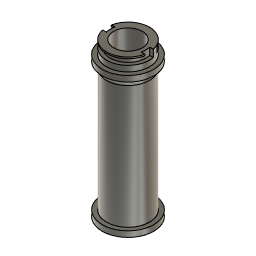
Spool_Holder_Handle_Easier_print_v1 (Autodesk Fusion 360 design; units mm, degrees)
Autodesk Fusion 360 part; units mm, degrees
sketch "Sketch1" plane through (0, 0, 0) normal (0, 0, 1) x (1, 0, 0)
  circle A0 centre (0, 0) radius 18
  dimension "d1" = 36
  constraint coincident A0.centre origin
  measures "d1" diameter of A0
sketch "Sketch2" plane through (0, 0, 0) normal (0, 0, 1) x (1, 0, 0)
  circle A0 centre (0, 0) radius 15
  circle A1 centre (0, 0) radius 13
  constraint coincident A0.centre A1.centre
extrude "Extrude1" add sketch "Sketch1" along normal blind 4
extrude "Extrude2" add sketch "Sketch2" along normal blind 110
sketch "Sketch3" plane through (0, 0, 110) normal (0, 0, 1) x (-1, 0, 0)
  circle A0 centre (0, 0) radius 15
  arc A1 (14.6969, 3) -> (3, 14.6969) centre (0, 0) ccw
  arc A2 (-3, 14.6969) -> (-14.6969, 3) centre (0, 0) ccw
  arc A3 (-14.6969, -3) -> (-3, -14.6969) centre (0, 0) ccw
  arc A4 (3, -14.6969) -> (14.6969, -3) centre (0, 0) ccw
  line L0 (11.619, -3) -> (14.6969, -3)
  arc A5 (11.619, -3) -> (11.619, 3) centre (0, 0) ccw
  arc A6 (3, 11.619) -> (-3, 11.619) centre (0, 0) ccw
  arc A7 (-11.619, 3) -> (-11.619, -3) centre (0, 0) ccw
  arc A8 (-3, -11.619) -> (3, -11.619) centre (0, 0) ccw
  line L1 (-14.6969, -3) -> (-11.619, -3)
  line L2 (14.6969, 3) -> (11.619, 3)
  line L3 (-11.619, 3) -> (-14.6969, 3)
  line L4 (-3, 14.6969) -> (-3, 11.619)
  line L5 (-3, -11.619) -> (-3, -14.6969)
  line L6 (3, -14.6969) -> (3, -11.619)
  line L7 (3, 11.619) -> (3, 14.6969)
  line L8 (8.6603, -5) -> (10.3923, -6)
  line L9 (0, 0) -> (12, 0) construction
  line L10 (-8.6603, -5) -> (-10.3923, -6)
  line L11 (4.8249, -8.3569) -> (6, -10.3923)
  line L12 (-4.8249, -8.3569) -> (-6, -10.3923)
  line L13 (8.6603, 5) -> (10.3923, 6)
  line L14 (-8.6603, 5) -> (-10.3923, 6)
  line L15 (5, 8.6603) -> (6, 10.3923)
  line L16 (-5, 8.6603) -> (-6, 10.3923)
  arc A9 (6, -10.3923) -> (10.3923, -6) centre (0, 0) ccw
  arc A10 (-3, -11.619) -> (3, -11.619) centre (0, 0) ccw
  arc A11 (-10.3923, -6) -> (-6, -10.3923) centre (0, 0) ccw
  arc A12 (-6, 10.3923) -> (-10.3923, 6) centre (0, 0) ccw
  arc A13 (3, 11.619) -> (-3, 11.619) centre (0, 0) ccw
  arc A14 (11.619, -3) -> (11.619, 3) centre (0, 0) ccw
  arc A15 (10.3923, 6) -> (6, 10.3923) centre (0, 0) ccw
  arc A16 (5, 8.6603) -> (-5, 8.6603) centre (0, 0) ccw
  arc A17 (-8.6603, 5) -> (-8.6603, -5) centre (0, 0) ccw
  arc A18 (-4.8249, -8.3569) -> (4.8249, -8.3569) centre (0, 0) ccw
  arc A19 (8.6603, -5) -> (8.6603, 5) centre (0, 0) ccw
  dimension "d6" = 30
  constraint coincident A4.start A1
  constraint perpendicular L1 L4
  constraint perpendicular L2 L4
  constraint concentric A1 A2
  constraint concentric A2 A3
  constraint concentric A3 A4
  constraint collinear L0 L1
  constraint coincident A6.start L6
  constraint concentric A5 A6
  constraint coincident A7.start L2
  constraint concentric A6 A7
  constraint coincident A8.start L4
  constraint concentric A7 A8
  constraint collinear L4 L5
  constraint collinear L6 L7
  constraint concentric A2 A16
  constraint concentric A7 A14
  constraint horizontal L9
  constraint coincident A0.centre A1.centre
  constraint coincident L10.end A14
  constraint coincident L11.end A14
  constraint perpendicular L10 L11
  constraint perpendicular L8 L12
  constraint coincident L13.end A14
  constraint parallel L10 L13
  constraint perpendicular L14 L15
  constraint coincident L16.end A14
  constraint concentric A9 A14
  constraint concentric A10 A14
  constraint concentric A11 A14
  constraint concentric A12 A14
  constraint concentric A13 A14
  constraint concentric A14 A15
  constraint concentric A16 A17
  constraint concentric A17 A18
  constraint concentric A18 A19
  measures "d6" angle of L8 L9
extrude "Extrude3" cut 1 faces at (14.2775, -0.7452, 110) along direction (0, 0, -1) blind 3
ref_plane "WorkPlane1" through (0, 0, 94) normal (0, 0, 1) x (1, 0, 0)
sketch "Sketch4" plane through (0, 0, 94) normal (0, 0, 1) x (1, 0, 0)
  circle A0 centre (0, 0) radius 18
  circle A1 centre (0, 0) radius 13
  constraint coincident A0.centre A1.centre
extrude "Extrude4" add sketch "Sketch4" along normal blind 4
sketch "Sketch5" plane through (0, 0, 94) normal (0, 0, 1) x (1, 0, 0)
  circle A0 centre (0, 0) radius 10
  circle A1 centre (0, 0) radius 15
  dimension "d12" = 20
  constraint coincident A0.centre A1.centre
  constraint concentric A0 A1
  measures "d12" diameter of A0
extrude "Extrude5" add sketch "Sketch5" along normal blind 13
ref_plane "WorkPlane2" through (0, 0, 102) normal (0, 0, 1) x (1, 0, 0)
sketch "Sketch6" plane through (0, 0, 102) normal (0, 0, 1) x (1, 0, 0)
  circle A0 centre (0, 0) radius 18
  line L0 (15, 3) -> (15, 7)
  line L1 (15, 7) -> (10.3562, 7)
  line L2 (15, 3) -> (12.1347, 3)
  line L3 (-15, -3) -> (-15, -7)
  line L4 (-15, -7) -> (-10.3562, -7)
  line L5 (-15, -3) -> (-12.1347, -3)
  arc A1 (-10.3562, -7) -> (12.1347, 3) centre (0, 0) ccw
  arc A2 (10.3562, 7) -> (-12.1347, -3) centre (0, 0) ccw
  dimension "d17" = 25
  dimension "d18" = 4
  dimension "d19" = 4
  constraint coincident A0.centre A1.centre
  constraint coincident L1.end A1
  constraint perpendicular L0 L1
  constraint perpendicular L3 L4
  constraint concentric A1 A2
  measures "d17" diameter of A1
  measures "d18" distance of L0.start L0.end
  measures "d19" distance of L3.start L3.end
extrude "Extrude6" cut sketch "Sketch6" along normal blind 4
sketch "Sketch7" plane through (0, 0, 107) normal (0, 0, 1) x (-1, 0, 0)
  circle A0 centre (0, 0) radius 10
  circle A1 centre (0, 0) radius 15
  line L0 (15, 3) -> (15, -3)
  line L1 (15, -3) -> (12.1347, -3)
  line L2 (15, 3) -> (12.1347, 3)
  line L3 (-15, 3) -> (-15, -3)
  line L4 (-15, -3) -> (-12.1347, -3)
  line L5 (-15, 3) -> (-12.1347, 3)
  arc A2 (12.1347, -3) -> (12.1347, 3) centre (0, 0) ccw
  arc A3 (-12.1347, 3) -> (-12.1347, -3) centre (0, 0) ccw
  dimension "d22" = 25
  dimension "d25" = 6
  constraint concentric A0 A2
  constraint perpendicular L0 L1
  constraint perpendicular L0 L2
  constraint perpendicular L3 L4
  constraint coincident L5.end A2
  constraint perpendicular L3 L5
  constraint concentric A2 A3
  measures "d22" diameter of A2
  measures "d25" distance of L3.start L3.end
extrude "Extrude7" cut sketch "Sketch7" against normal blind 2 contours A1 L1 L2 A2 | A1 L4 L5 A3
sketch "Sketch8" plane through (0, 0, 107) normal (0, 0, 1) x (-1, 0, 0)
  line L0 (14.6969, -3) -> (12.1347, -3)
  arc A0 (12.1347, -3) -> (12.1347, 3) centre (0, 0) ccw
  line L1 (12.1347, 3) -> (14.6969, 3)
  arc A1 (14.6969, 3) -> (-14.6969, 3) centre (0, 0) ccw
  line L2 (-14.6969, 3) -> (-12.1347, 3)
  arc A2 (-12.1347, 3) -> (-12.1347, -3) centre (0, 0) ccw
  line L3 (-12.1347, -3) -> (-14.6969, -3)
  arc A3 (-14.6969, -3) -> (14.6969, -3) centre (0, 0) ccw
  circle A4 centre (0, 0) radius 10
  line L4 (9, 9.5) -> (9, 8.6747)
  line L5 (9, 9.5) -> (8.124, 9.5)
  line L6 (0, 0) -> (13.086, 0) construction
  line L7 (-9, -9.5) -> (-9, -8.6747)
  line L8 (-9, -9.5) -> (-8.124, -9.5)
  arc A5 (-9, -8.6747) -> (-8.124, -9.5) centre (0, 0) ccw
  arc A6 (9, 8.6747) -> (8.124, 9.5) centre (0, 0) ccw
  constraint perpendicular L4 L5
  constraint coincident A0.centre A1.centre
  constraint horizontal L6
  constraint vertical L7
  constraint perpendicular L7 L8
extrude "Extrude8" add sketch "Sketch8" against normal blind 5 contours L4 L5 A6 | L7 L8 A5
fillet "Fillet1" radius 0.35 1 edges at (9, 9.5, 104)
fillet "Fillet2" radius 0.35 1 edges at (-9, -9.5, 104)
fillet "Fillet3" radius 1.5 2 edges at (-9, -8.6747, 104) (-8.124, -9.5, 104)
fillet "Fillet4" radius 1.5 2 edges at (8.124, 9.5, 104) (9, 8.6747, 104)
extrude "Extrude9" add 1 faces at (11.9516, 0.6458, 94) along direction (0, 0, -1) blind 8
fillet "Fillet5" radius 4.5 1 edges at (-13.9849, 5.4242, 94)
fillet "Fillet6" radius 0.65 6 edges at (-4.0593, 11.8225, 106) (8.1644, 9.5843, 106) (8.651, 9.5, 106) (8.8904, 9.4043, 106) (9.1105, 8.6905, 106) (9.8845, 7.6516, 106)
fillet "Fillet7" radius 12.25 1 edges at (-12.1203, -4.701, 86)
fillet "Fillet8" radius 0.65 6 edges at (4.0593, -11.8225, 106) (-8.1644, -9.5843, 106) (-8.651, -9.5, 106) (-8.8904, -9.4043, 106) (-9.1105, -8.6905, 106) (-9.8845, -7.6516, 106)
